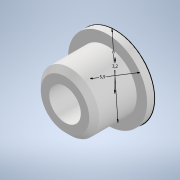
# Autodesk Inventor part: middle_gear_fixator
Saved by Autodesk Inventor 2022 (Build 260153000, 153)
## iProperties
Created: 2024-09-10
Part Number: middle_gear_fixator
Material: Типовые
Document SubType Name: Modeling
Designer: Andrey
Density: 1 g/cm^3
Appearance: По умолчанию
Author: Andrey
Autodesk Inventor part; units mm, degrees
ref_plane "YZ Plane" through (0, 0, 0) normal (1, 0, 0) x (0, 1, 0)
ref_plane "XZ Plane" through (0, 0, 0) normal (0, 1, 0) x (-1, 0, 0)
ref_plane "XY Plane" through (0, 0, 0) normal (0, 0, 1) x (1, 0, 0)
sketch "Эскиз1" plane through (0, 0, 0) normal (0, 0, 1) x (1, 0, 0)
  circle A0 centre (0, 0) radius 2.95
  circle A1 centre (0, 0) radius 1.6
  circle A2 centre (0, 0) radius 4
  dimension "d0" = 5.9
  dimension "d1" = 3.2
  dimension "d2" = 8
  constraints: 3 centre point, 3 coincident
  measures "d0" diameter of A0
  measures "d1" diameter of A1
  measures "d2" diameter of A2
sketch "Эскиз2" plane through (0, 0, 0) normal (0, 0, 1) x (1, 0, 0)
  circle A0 centre (0, 0) radius 2.95 projected
  circle A1 centre (0, 0) radius 1.6 projected
  circle A2 centre (0, 0) radius 4 projected
extrude "Выдавливание1" add sketch "Эскиз2" along normal blind 0.75 contours A0 | A2
sketch "Эскиз4" plane through (0, 0, 0.75) normal (0, 0, 1) x (1, 0, 0)
  circle A0 centre (0, 0) radius 2.95
  circle A1 centre (0, 0) radius 1.6 projected
  dimension "d7" = 5.9
  constraints: 1 centre point, 1 coincident
  measures "d7" diameter of A0
extrude "Выдавливание3" add sketch "Эскиз4" along normal blind 4.3
chamfer "Фаска1" distance 0.5 angle 45 1 edges at (-2.95, 0, 5.05)
